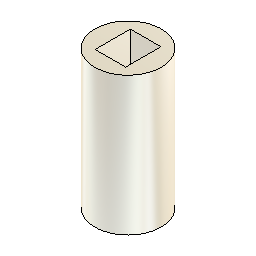
MC ES Coupler TII (Autodesk Fusion 360 design; units mm, degrees)
Autodesk Fusion 360 part; units mm, degrees
sketch "Sketch1" plane through (0, 0, 0) normal (0, 0, 1) x (1, 0, 0)
  line L0 (5.52, 3.187) -> (0, 6.3739)
  line L1 (0, 6.3739) -> (-5.52, 3.187)
  line L2 (-5.52, 3.187) -> (-5.52, -3.187)
  line L3 (-5.52, -3.187) -> (0, -6.3739)
  line L4 (0, -6.3739) -> (5.52, -3.187)
  line L5 (5.52, -3.187) -> (5.52, 3.187)
  circle A0 centre (0, 0) radius 12
  line L6 (-2.76, 4.7805) -> (-6, 10.3923) construction
  line L7 (2.76, -4.7805) -> (6, -10.3923) construction
  line L8 (0, -6.3739) -> (-5.52, -6.3739)
  line L9 (-5.52, -6.3739) -> (-5.52, -3.187)
  line L10 (0, -6.3739) -> (5.52, -6.3739)
  line L11 (5.52, -6.3739) -> (5.52, -3.187)
  line L12 (5.52, 3.187) -> (5.52, 6.3739)
  line L13 (5.52, 6.3739) -> (0, 6.3739)
  line L14 (-5.52, 3.187) -> (-5.52, 6.3739)
  line L15 (-5.52, 6.3739) -> (0, 6.3739)
  dimension "d1" = 5.52
  dimension "d2" = 24
  constraint coincident A0.centre origin
  constraint midpoint L1 L6.start
  constraint coincident A0 L6.end
  constraint perpendicular L1 L6
  constraint midpoint L4 L7.start
  constraint coincident A0 L7.end
  constraint perpendicular L4 L7
  constraint perpendicular L2 L8
  constraint perpendicular L8 L9
  constraint perpendicular L5 L10
  constraint perpendicular L8 L11
  constraint parallel L5 L12
  constraint perpendicular L5 L13
  constraint perpendicular L13 L14
  constraint perpendicular L14 L15
  measures "d1" distance of A0.centre L5
  measures "d2" diameter of A0
extrude "Extrude1" add sketch "Sketch1" along normal blind 38 and the other way blind 12 contours L0 L1 L2 L3 L4 L5 | L0 L12 L13 | L1 L14 L15 | L4 L10 L11 | L3 L8 L9 | A0
extrude "Extrude2" cut sketch "Sketch1" along normal blind 35 from surface at 3 contours L0 L1 L2 L3 L4 L5 | L0 L12 L13 | L1 L14 L15 | L4 L10 L11 | L3 L8 L9
named bodies: "Coupler"
